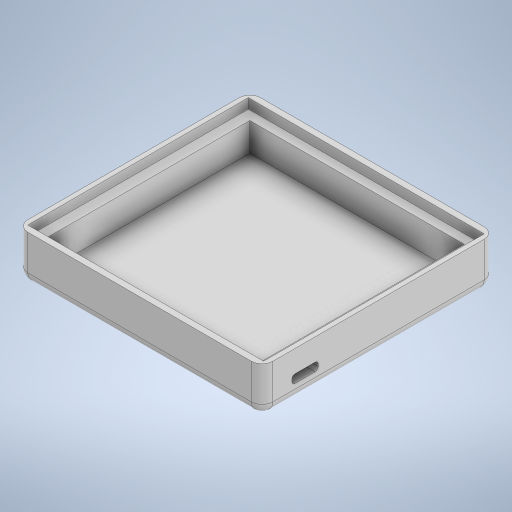
# Autodesk Inventor part: backdoor
Saved by Autodesk Inventor 2023.6 (Build 276521000, 521)
## iProperties
Created: 2026-05-31
Part Number: backdoor
Material: Generic
Document SubType Name: Modeling
Designer: Nanda
Density: 1 g/cm^3
Appearance: Default
Author: Nanda
Autodesk Inventor part; units mm, degrees
ref_plane "YZ Plane" through (0, 0, 0) normal (1, 0, 0) x (0, 1, 0)
ref_plane "XZ Plane" through (0, 0, 0) normal (0, 1, 0) x (-1, 0, 0)
ref_plane "XY Plane" through (0, 0, 0) normal (0, 0, 1) x (1, 0, 0)
sketch "Sketch2" plane through (0, 0, 0) normal (0, 1, 0) x (-1, 0, 0)
  line L0 (-40, -38) -> (40, -38)
  line L1 (40, -38) -> (40, 38)
  line L2 (40, 38) -> (-40, 38)
  line L3 (-40, 38) -> (-40, -38)
  line L4 (-40, -38) -> (40, 38) construction
  line L5 (40, -38) -> (-40, 38) construction
  point P0 (0, 0)
  dimension "d0" = 80
  dimension "d1" = 76
  constraints: 12 end point, 2 midpoint, 2 parallel, 1 horizontal, 1 perpendicular
  measures "d0" distance of L2.end L1.end
  measures "d1" distance of L1.end L0.end
extrude "Extrusion1" add sketch "Sketch2" along normal blind 2.5
sketch "Sketch3" plane through (0, 2.5, 0) normal (0, 1, 0) x (1, 0, 0)
  line L0 (-35, -33) -> (35, -33)
  line L1 (35, -33) -> (35, 33)
  line L2 (35, 33) -> (-35, 33)
  line L3 (-35, 33) -> (-35, -33)
  line L4 (-35, -33) -> (35, 33) construction
  line L5 (35, -33) -> (-35, 33) construction
  line L6 (-40, 38) -> (-40, -38) projected
  line L7 (-40, 38) -> (-40, -38) projected
  line L8 (-40, -38) -> (40, -38) projected
  line L9 (-40, -38) -> (40, -38) projected
  line L10 (40, -38) -> (40, 38) projected
  line L11 (40, -38) -> (40, 38) projected
  line L12 (40, 38) -> (-40, 38) projected
  line L13 (40, 38) -> (-40, 38) projected
  point P0 (0, 0)
  dimension "d4" = 70
  dimension "d5" = 66
  constraints: 12 end point, 2 midpoint, 2 parallel, 1 horizontal, 1 perpendicular
  measures "d4" distance of L2.end L1.end
  measures "d5" distance of L1.end L0.end
extrude "Extrusion2" add sketch "Sketch3" along normal blind 12.5
sketch "Sketch4" plane through (40, 0, 38) normal (1, 0, 0) x (0, 0, -1)
  line L0 (76, 0) -> (0, 0) projected
  line L1 (0, 0) -> (0, 15) projected
  line L2 (76, 0) -> (76, 15) projected
  line L3 (71, 2.5) -> (71, 15) projected
  line L4 (76, 15) -> (0, 15) projected
  line L5 (71, 2.5) -> (5, 2.5) projected
  line L6 (5, 2.5) -> (5, 15) projected
  line L7 (5, 15) -> (71, 15) projected
  line L8 (71, 15) -> (5, 15) projected
  line L9 (5, 2.5) -> (71, 2.5) projected
  line L10 (5, 2.5) -> (5, 15) projected
  line L11 (0, 0) -> (0, 15) projected
  line L12 (0, 0) -> (76, 0) projected
  line L13 (0, 15) -> (76, 15) projected
  line L14 (71, 2.5) -> (71, 15) projected
  line L15 (76, 0) -> (76, 15) projected
  line L16 (10.7, 5.15) -> (17.3, 5.15)
  line L17 (18.3, 6.15) -> (18.3, 6.85)
  line L18 (17.3, 7.85) -> (10.7, 7.85)
  line L19 (9.7, 6.85) -> (9.7, 6.15)
  line L20 (9.7, 5.15) -> (18.3, 7.85) construction
  line L21 (18.3, 5.15) -> (9.7, 7.85) construction
  arc A0 (18.3, 6.85) -> (17.3, 7.85) centre (17.3, 6.85) ccw
  arc A1 (17.3, 5.15) -> (18.3, 6.15) centre (17.3, 6.15) ccw
  arc A2 (10.7, 7.85) -> (9.7, 6.85) centre (10.7, 6.85) ccw
  arc A3 (9.7, 6.15) -> (10.7, 5.15) centre (10.7, 6.15) ccw
  point P0 (38, 0)
  point P1 (14, 6.5)
  dimension "d8" = 8.6
  dimension "d9" = 2.7
  dimension "d10" = 1
  dimension "d11" = 1
  dimension "d12" = 4
  dimension "d13" = 9
  constraints: 12 end point, 8 point on circle, 8 point on line, 8 tangent, 4 centre point, 2 equal radius, 2 midpoint, 2 parallel, 1 horizontal, 1 perpendicular
  measures "d8" distance of L21.end L20.end
  measures "d9" distance of L20.end L21.start
  measures "d10" radius of A0
  measures "d11" radius of A1
  measures "d12" distance from line of L5 point (14, 6.5)
  measures "d13" distance from line of L10 point (14, 6.5)
extrude "Extrusion3" cut sketch "Sketch4" against normal blind 12.5 contours A3 L19 A2 L18 A0 L17 A1 L16
fillet "Fillet1" radius 3.5 8 edges at (40, 7.5, -38) (40, 7.5, 38) (-40, 7.5, 38) (-40, 7.5, -38) (-40, 0, 0) (0, 0, -38) (40, 0, 0) (0, 0, 38)
sketch "Sketch5" plane through (0, 15, 0) normal (0, 1, 0) x (1, 0, 0)
  line L0 (36.5, 38) -> (-36.5, 38) projected
  line L1 (-36.5, -38) -> (36.5, -38) projected
  line L2 (40, -34.5) -> (40, 34.5) projected
  line L3 (-40, 34.5) -> (-40, -34.5) projected
  line L4 (35, -33) -> (-35, -33) projected
  line L5 (-35, -33) -> (-35, 33) projected
  line L6 (-35, 33) -> (35, 33) projected
  line L7 (35, 33) -> (35, -33) projected
  line L8 (-38.5, -36) -> (38.5, -36)
  line L9 (38.5, -36) -> (38.5, 36)
  line L10 (38.5, 36) -> (-38.5, 36)
  line L11 (-38.5, 36) -> (-38.5, -36)
  line L12 (-38.5, -36) -> (38.5, 36) construction
  line L13 (38.5, -36) -> (-38.5, 36) construction
  point P0 (0, 0)
  dimension "d17" = 76
  dimension "d18" = 80
  dimension "d19" = 77
  dimension "d20" = 72
  constraints: 12 end point, 2 midpoint, 2 parallel, 1 horizontal, 1 perpendicular
  measures "d17" distance between parallel lines of L0 L1
  measures "d18" distance between parallel lines of L2 L3
  measures "d19" distance of L10.end L9.end
  measures "d20" distance of L9.end L8.end
extrude "Extrusion4" cut sketch "Sketch5" against normal blind 3.2
body "Solid1"
